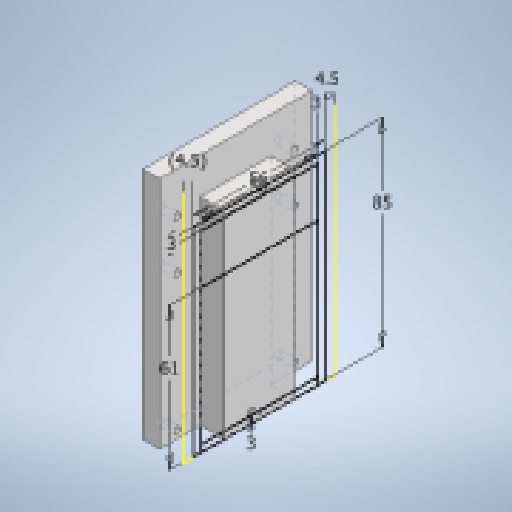
# Autodesk Inventor part: pi_holder
Saved by Autodesk Inventor 2023 (Build 270158000, 158)
## iProperties
Created: 2022-10-03
Part Number: pi_holder
Material: Generic
Document SubType Name: Modeling
Designer: carso
Density: 1 g/cm^3
Appearance: Default
Author: carso
Autodesk Inventor part; units mm, degrees
ref_plane "YZ Plane" through (0, 0, 0) normal (1, 0, 0) x (0, 1, 0)
ref_plane "XZ Plane" through (0, 0, 0) normal (0, 1, 0) x (-1, 0, 0)
ref_plane "XY Plane" through (0, 0, 0) normal (0, 0, 1) x (1, 0, 0)
sketch "Sketch1" plane through (0, 0, 0) normal (0, 0, 1) x (1, 0, 0)
  line L0 (0, 0) -> (-25, 0)
  line L1 (-25, 0) -> (-25, 100)
  line L2 (-25, 100) -> (0, 100)
  line L3 (0, 100) -> (0, 0)
  line L4 (0, 0) -> (-18, 0)
  line L5 (-18, 0) -> (-18, 85)
  line L6 (0, 85) -> (0, 0)
  line L7 (0, 85) -> (0, 65)
  line L8 (-18, 85) -> (-18, 100)
  point P0 (-18, 0)
  point P1 (-18, 92.5)
  dimension "d0" = 25
  dimension "d1" = 100
  dimension "d6" = 20
  dimension "d78" = 7
  constraints: 18 end point, 3 parallel, 3 perpendicular, 2 horizontal, 2 point on line, 1 midpoint
  measures "d0" distance of L1.end L2.end
  measures "d1" distance of L0.end L1.end
  measures "d6" distance of L6.start L7.end
  measures "d78" distance from line of L1 point (-18, 92.5)
extrude "Extrusion1" add sketch "Sketch1" along normal blind 65 contours L0 L1 L2 L8 L5
sketch "Sketch2" plane through (-18, 0, 0) normal (1, 0, 0) x (0, 0, -1)
  line L0 (0, 0) -> (-65, 0) projected
  line L1 (0, 100) -> (-65, 100) projected
  line L2 (-47.5, 0) -> (-17.5, 0)
  line L3 (-17.5, 0) -> (-17.5, 100)
  line L4 (-17.5, 100) -> (-47.5, 100)
  line L5 (-47.5, 100) -> (-47.5, 0)
  line L6 (-65, 0) -> (-65, 100) projected
  line L7 (0, 0) -> (0, 100) projected
  line L8 (-47.5, 84.5192) -> (-17.5, 84.5192)
  dimension "d8" = 30
  dimension "d9" = 17.5
  dimension "d10" = 17.5
  constraints: 10 end point, 4 point on line, 2 parallel, 2 perpendicular, 1 horizontal
  measures "d8" distance of L4.end L3.end
  measures "d9" distance between parallel lines of L5 L6
  measures "d10" distance between parallel lines of L7 L3
extrude "Extrusion2" add sketch "Sketch2" along normal blind 10 contours L0 L5 L8 L3
sketch "Sketch6" plane through (-8, 0, 0) normal (1, 0, 0) x (0, 0, -1)
  line L0 (0, 0) -> (-65, 0) projected
  line L1 (-60.5, 0) -> (-4.5, 0)
  line L2 (-4.5, 0) -> (-4.5, 85)
  line L3 (-4.5, 85) -> (-60.5, 85)
  line L4 (-60.5, 85) -> (-60.5, 0)
  line L5 (0, 0) -> (0, 100) projected
  line L6 (-65, 0) -> (-65, 100) projected
  line L7 (-57.5, 0) -> (-7.5, 0)
  line L8 (-7.5, 0) -> (-7.5, 82)
  line L9 (-7.5, 82) -> (-57.5, 82)
  line L10 (-57.5, 82) -> (-57.5, 0)
  line L11 (-57.5, 61) -> (-7.5, 61)
  line L12 (-57.5, 3) -> (-7.5, 3)
  point P0 (-32.5, 3)
  dimension "d27" = 56
  dimension "d28" = 85
  dimension "d29" = 4.5
  dimension "d30" = 4.5
  dimension "d31" = 50
  dimension "d32" = 3
  dimension "d33" = 3
  dimension "d34" = 61
  dimension "d49" = 3
  constraints: 20 end point, 6 point on line, 4 parallel, 4 perpendicular, 2 horizontal, 1 midpoint
  measures "d27" distance of L3.end L2.end
  measures "d28" distance of L3.end L1.start
  measures "d29" distance between parallel lines of L5 L2
  measures "d30" distance between parallel lines of L4 L6
  measures "d31" distance of L9.end L8.end
  measures "d32" distance between parallel lines of L3 L9
  measures "d33" distance between parallel lines of L2 L8
  measures "d34" distance between parallel lines of L0 L11
  measures "d49" distance from line of L0 point (-32.5, 3)
hole "Hole3" at (-8, 61, 7.5) direction (-1, 0, 0) diameter 3 depth 40
hole "Hole4" at (-8, 82, 7.5) direction (-1, 0, 0) diameter 3 depth 40
hole "Hole5" at (-8, 3, 7.5) direction (-1, 0, 0) diameter 3 depth 40
hole "Hole6" at (-8, 3, 57.5) direction (-1, 0, 0) diameter 3 depth 40
hole "Hole7" at (-8, 61, 57.5) direction (-1, 0, 0) diameter 3 depth 40
hole "Hole8" at (-8, 82, 57.5) direction (-1, 0, 0) diameter 3 depth 40
fillet "Fillet1" radius 2 1 edges at (-8, 84.5192, 32.5)
body "Solid1"
